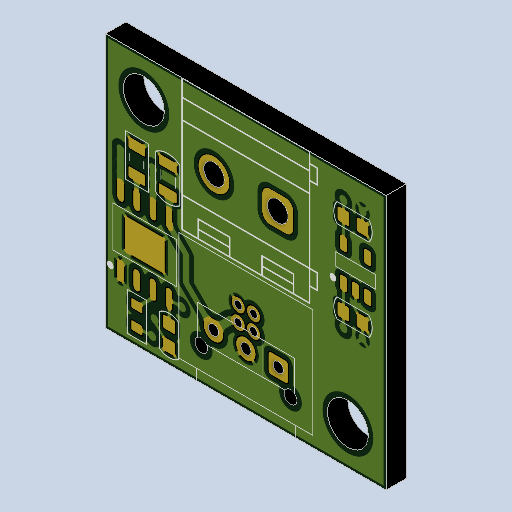
# Autodesk Inventor part: valve_driver_BOARD
Saved by Autodesk Inventor 2025.4 (Build 294407000, 407)
## iProperties
Created: 2025-07-29
Part Number: valve_driver_BOARD
Material: Generic
Document SubType Name: Modeling
Designer: Yuhsuan Chen
Density: 1 g/cm^3
Appearance: BoardColor
Author: Yuhsuan Chen
Autodesk Inventor part; units mm, degrees
ref_plane "YZ Plane" through (0, 0, 0) normal (1, 0, 0) x (0, 1, 0)
ref_plane "XZ Plane" through (0, 0, 0) normal (0, 1, 0) x (-1, 0, 0)
ref_plane "BoardFrontPlane" through (0, 0, 0) normal (0, 0, 1) x (1, 0, 0)
sketch "Sketch1" plane through (0, 0, 0) normal (0, 0, 1) x (1, 0, 0)
  line L0 (161.6857, 93.5857) -> (161.6857, 113.5857)
  line L1 (161.6857, 113.5857) -> (183.6857, 113.5857)
  line L2 (183.6857, 113.5857) -> (183.6857, 93.5857)
  line L3 (183.6857, 93.5857) -> (161.6857, 93.5857)
  constraints: 8 end point
extrude "BoardOutline" add sketch "Sketch1" along normal blind 1.5954
sketch "Sketch10" plane through (0, 0, 1.5954) normal (0, 0, 1) x (1, 0, 0)
  point P0 (175.1857, 108.2857)
hole "CN3-1" at (175.1857, 108.2857, 1.5954) direction (0, 0, -1) diameter 1.6 end through all
sketch "Sketch11" plane through (0, 0, 1.5954) normal (0, 0, 1) x (1, 0, 0)
  point P0 (170.1857, 108.2857)
hole "CN3-2" at (170.1857, 108.2857, 1.5954) direction (0, 0, -1) diameter 1.6 end through all
sketch "Sketch12" plane through (0, 0, 1.5954) normal (0, 0, 1) x (1, 0, 0)
  point P0 (164.6857, 110.5857)
hole "Free-1" at (164.6857, 110.5857, 1.5954) direction (0, 0, -1) diameter 3.2 end through all
sketch "Sketch13" plane through (0, 0, 1.5954) normal (0, 0, 1) x (1, 0, 0)
  point P0 (180.6857, 96.5857)
hole "Free-0" at (180.6857, 96.5857, 1.5954) direction (0, 0, -1) diameter 3.2 end through all
sketch "img_Top" plane through (0, 0, 1.5954) normal (0, 0, 1) x (1, 0, 0)
  line L0 (161.6857, 113.5857) -> (183.6857, 113.5857) construction
  line L1 (183.6857, 113.5857) -> (183.6857, 93.5926) construction
  line L2 (183.6857, 93.5926) -> (161.6857, 93.5926) construction
  line L3 (161.6857, 93.5926) -> (161.6857, 113.5857) construction
  constraints: 2 other
decal "Decal_Top"
sketch "img_Bottom" plane through (0, 0, -1.5954) normal (0, 0, -1) x (1, 0, 0)
  line L0 (161.6857, -93.5857) -> (183.6857, -93.5857) construction
  line L1 (183.6857, -93.5857) -> (183.6857, -113.5787) construction
  line L2 (183.6857, -113.5787) -> (161.6857, -113.5787) construction
  line L3 (161.6857, -113.5787) -> (161.6857, -93.5857) construction
  constraints: 2 other
decal "Decal_Bottom"
sketch "Sketch16" plane through (0, 0, 1.5954) normal (0, 0, 1) x (1, 0, 0)
  point P0 (172.0857, 99.1607)
hole "CN2-4" at (172.0857, 99.1607, 1.5954) direction (0, 0, -1) diameter 0.6 end through all
sketch "Sketch17" plane through (0, 0, 1.5954) normal (0, 0, 1) x (1, 0, 0)
  point P0 (172.0857, 100.3607)
hole "CN2-1" at (172.0857, 100.3607, 1.5954) direction (0, 0, -1) diameter 0.6 end through all
sketch "Sketch18" plane through (0, 0, 1.5954) normal (0, 0, 1) x (1, 0, 0)
  point P0 (173.2857, 99.1607)
hole "CN2-3" at (173.2857, 99.1607, 1.5954) direction (0, 0, -1) diameter 0.6 end through all
sketch "Sketch19" plane through (0, 0, 1.5954) normal (0, 0, 1) x (1, 0, 0)
  point P0 (173.2857, 100.3607)
hole "CN2-2" at (173.2857, 100.3607, 1.5954) direction (0, 0, -1) diameter 0.6 end through all
sketch "Sketch20" plane through (0, 0, 1.5954) normal (0, 0, 1) x (1, 0, 0)
  point P0 (169.1857, 96.1607)
hole "CN2-0_SEOGABLU" at (169.1857, 96.1607, 1.5954) direction (0, 0, -1) diameter 1 end through all
sketch "Sketch21" plane through (0, 0, 1.5954) normal (0, 0, 1) x (1, 0, 0)
  point P0 (176.1857, 96.1607)
hole "CN2-0_AERYPNHJ" at (176.1857, 96.1607, 1.5954) direction (0, 0, -1) diameter 1 end through all
sketch "Sketch22" plane through (0, 0, 1.5954) normal (0, 0, 1) x (1, 0, 0)
  point P0 (172.6857, 97.6857)
hole "CN1-2" at (172.6857, 97.6857, 1.5954) direction (0, 0, -1) diameter 0.8 end through all
sketch "Sketch23" plane through (0, 0, 1.5954) normal (0, 0, 1) x (1, 0, 0)
  point P0 (170.1457, 97.6857)
hole "CN1-3" at (170.1457, 97.6857, 1.5954) direction (0, 0, -1) diameter 0.8 end through all
sketch "Sketch24" plane through (0, 0, 1.5954) normal (0, 0, 1) x (1, 0, 0)
  point P0 (175.2257, 97.6857)
hole "CN1-1" at (175.2257, 97.6857, 1.5954) direction (0, 0, -1) diameter 0.8 end through all
body "Solid1"
